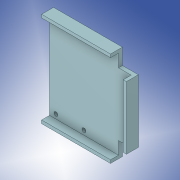
# Autodesk Inventor part: BB001
Saved by Autodesk Inventor 2017 SP1 (Build 210196100, 196)
## iProperties
Created: 2017-08-08
Part Number: BB001
Material: ABS Plastic
Document SubType Name: Modeling
Designer: Zach
Density: 1.06 g/cm^3
Appearance: CR Light Blue
Author: Zach
Autodesk Inventor part; units mm, degrees
ref_plane "YZ Plane" through (0, 0, 0) normal (1, 0, 0) x (0, 1, 0)
ref_plane "XZ Plane" through (0, 0, 0) normal (0, 1, 0) x (-1, 0, 0)
ref_plane "XY Plane" through (0, 0, 0) normal (0, 0, 1) x (1, 0, 0)
sketch "Sketch1" plane through (0, 0, 0) normal (0, 0, 1) x (1, 0, 0)
  line L0 (0, 0) -> (106.5, 0) construction
  line L1 (106.5, 0) -> (106.5, 119) construction
  line L2 (106.5, 119) -> (0, 119) construction
  line L3 (0, 119) -> (0, 0) construction
  line L4 (106.5, 119) -> (86.5, 119) construction
  line L5 (86.5, 119) -> (86.5, 99) construction
  line L6 (86.5, 99) -> (106.5, 99) construction
  line L7 (106.5, 99) -> (106.5, 119) construction
  line L8 (106.5, 0) -> (86.5, 0) construction
  line L9 (86.5, 0) -> (86.5, 20) construction
  line L10 (86.5, 20) -> (106.5, 20) construction
  line L11 (106.5, 20) -> (106.5, 0) construction
  line L12 (0, 119) -> (86.5, 119)
  line L13 (86.5, 119) -> (86.5, 99)
  line L14 (86.5, 99) -> (106.5, 99)
  line L15 (106.5, 20) -> (86.5, 20)
  line L16 (86.5, 0) -> (86.5, 20)
  line L17 (86.5, 0) -> (0, 0)
  line L18 (0, 0) -> (0, 119)
  line L19 (106.5, 99) -> (106.5, 20)
  dimension "d0" = 106.5
  dimension "d1" = 119
  dimension "d2" = 20
  dimension "d3" = 20
  dimension "d4" = 20
  dimension "d5" = 20
  constraints: 40 end point, 7 collinear, 6 parallel, 4 perpendicular, 3 horizontal
  measures "d0" distance of L2.end L1.end
  measures "d1" distance of L1.end L0.end
  measures "d2" distance of L6.end L5.end
  measures "d3" distance of L4.end L5.end
  measures "d4" distance of L9.end L10.end
  measures "d5" distance of L8.end L9.end
extrude "Extrusion1" add sketch "Sketch1" along normal blind 5
sketch "Sketch2" plane through (0, 0, 5) normal (0, 0, 1) x (1, 0, 0)
  circle A0 centre (43.25, 9.5) radius 2.5
  circle A1 centre (97, 59.5) radius 2.5
  circle A2 centre (43.25, 109.5) radius 2.5
  line L0 (86.5, 119) -> (0, 119) projected
  line L1 (0, 0) -> (86.5, 0) projected
  line L2 (106.5, 20) -> (106.5, 99) projected
  circle A3 centre (8, 109.5) radius 2.5
  circle A4 centre (8, 9.5) radius 2.5
  line L3 (0, 119) -> (0, 0) projected
  point P0 (106.5, 59.5)
  point P1 (43.25, 119)
  point P2 (43.25, 0)
  dimension "d8" = 5
  dimension "d9" = 5
  dimension "d10" = 5
  dimension "d11" = 9.5
  dimension "d12" = 9.5
  dimension "d13" = 9.5
  dimension "d21" = 5
  dimension "d22" = 5
  dimension "d23" = 8
  constraints: 5 centre point, 3 horizontal alignment, 3 midpoint, 3 vertical alignment
  measures "d8" diameter of A0
  measures "d9" diameter of A1
  measures "d10" diameter of A2
  measures "d11" distance from line of L0 A2.centre
  measures "d12" distance from line of L1 A0.centre
  measures "d13" distance from line of L2 A1.centre
  measures "d21" diameter of A3
  measures "d22" diameter of A4
  measures "d23" distance from line of L3 A3.centre
extrude "Extrusion2" cut sketch "Sketch2" against normal through all
sketch "Sketch3" plane through (0, 0, 5) normal (0, 0, 1) x (1, 0, 0)
  line L0 (86.5, 119) -> (0, 119) projected
  line L1 (86.5, 99) -> (86.5, 119) projected
  line L2 (106.5, 99) -> (86.5, 99) projected
  line L3 (106.5, 20) -> (106.5, 99) projected
  line L4 (86.5, 20) -> (106.5, 20) projected
  line L5 (86.5, 0) -> (86.5, 20) projected
  line L6 (0, 0) -> (86.5, 0) projected
  line L7 (0, 115) -> (82.5, 115)
  line L8 (82.5, 115) -> (82.5, 95)
  line L9 (82.5, 95) -> (102.5, 95)
  line L10 (102.5, 95) -> (102.5, 24)
  line L11 (102.5, 24) -> (82.5, 24)
  line L12 (82.5, 24) -> (82.5, 4)
  line L13 (82.5, 4) -> (0, 4)
  line L14 (0, 119) -> (0, 115)
  line L15 (0, 119) -> (0, 0) projected
  line L16 (0, 4) -> (0, 0)
  dimension "d16" = 4
  constraints: 18 end point, 2 collinear, 6 other
  measures "d16" distance between parallel lines of L0 L7
extrude "Extrusion3" add sketch "Sketch3" along normal blind 10 contours L1 L2 L3 L4 L5 L6 L15 L13 L12 L11 L10 L9 L8 L7 L14 L0
sketch "Sketch4" plane through (0, 0, 15) normal (0, 0, 1) x (1, 0, 0)
  line L0 (82.5, 115) -> (0, 115) projected
  line L1 (82.5, 115) -> (102.5, 115)
  line L2 (102.5, 115) -> (102.5, 4)
  line L3 (102.5, 4) -> (82.5, 4)
  line L4 (82.5, 4) -> (82.5, 115)
  point P0 (0, 0)
  point P1 (102.5, 95)
  constraints: 8 end point, 2 parallel, 1 horizontal, 1 horizontal alignment, 1 perpendicular, 1 vertical alignment
extrude "Extrusion4" cut sketch "Sketch4" against normal blind 10
body "Solid1"
